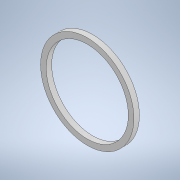
# Autodesk Inventor part: 4002_Bias_Coil_Holder_Tube_Mount_Layer3_MPSv2_v1
Saved by Autodesk Inventor 2021 (Build 250183000, 183)
## iProperties
Created: 2021-02-18
Part Number: 4002_Bias_Coil_Holder_Tube_Mount_Layer3_MPSv2_v1
Material: Generic
Document SubType Name: Modeling
Designer: Barksdale
Density: 1 g/cm^3
Appearance: Default
Author: Barksdale
Autodesk Inventor part; units mm, degrees
ref_plane "YZ Plane" through (0, 0, 0) normal (1, 0, 0) x (0, 1, 0)
ref_plane "XZ Plane" through (0, 0, 0) normal (0, 1, 0) x (-1, 0, 0)
ref_plane "XY Plane" through (0, 0, 0) normal (0, 0, 1) x (1, 0, 0)
sketch "Sketch1" plane through (0, 0, 0) normal (0, 0, 1) x (1, 0, 0)
  circle A0 centre (0, 0) radius 51.129
  circle A1 centre (0, 0) radius 45.0088
  dimension "d0" = 102.258
  dimension "d1" = 90.0176
  constraints: 2 centre point, 2 coincident
  measures "d0" diameter of A0
  measures "d1" diameter of A1
extrude "Extrusion1" add sketch "Sketch1" along normal blind 6
body "Solid1"
